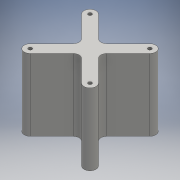
# Autodesk Inventor part: 60x60SlimSpacer
Saved by Autodesk Inventor 2016 (Build 200138000, 138)
## iProperties
Created: 2016-05-22
Part Number: 60x60SlimSpacer
Material: Generic
Document SubType Name: Modeling
Designer: Kurtis
Density: 1 g/cm^3
Appearance: Default
Author: Kurtis
Autodesk Inventor part; units mm, degrees
ref_plane "YZ Plane" through (0, 0, 0) normal (1, 0, 0) x (0, 1, 0)
ref_plane "XZ Plane" through (0, 0, 0) normal (0, 1, 0) x (-1, 0, 0)
ref_plane "XY Plane" through (0, 0, 0) normal (0, 0, 1) x (1, 0, 0)
sketch "Sketch1" plane through (0, 0, 0) normal (0, 0, 1) x (1, 0, 0)
  line L0 (-30, -30) -> (30, 30) construction
  line L1 (30, -30) -> (-30, 30) construction
  line L2 (25, 30) -> (25, 25) construction
  line L3 (-30, 30) -> (-25, 30) construction
  line L4 (-25, 30) -> (-25, 25) construction
  line L5 (-30, -25) -> (-25, -25) construction
  line L6 (30, -25) -> (25, -25) construction
  circle A0 centre (-25, 25) radius 1.5
  circle A1 centre (25, 25) radius 1.5
  circle A2 centre (25, -25) radius 1.5
  circle A3 centre (-25, -25) radius 1.5
  arc A4 (-21.4645, 28.5355) -> (-28.5355, 21.4645) centre (-25, 25) ccw
  arc A5 (28.5355, 21.4645) -> (21.4645, 28.5355) centre (25, 25) ccw
  arc A6 (21.4645, -28.5355) -> (28.5355, -21.4645) centre (25, -25) ccw
  arc A7 (-28.5355, -21.4645) -> (-21.4645, -28.5355) centre (-25, -25) ccw
  line L7 (-25, 25) -> (-30, 20) construction
  line L8 (-30, 20) -> (-20, 30) construction
  line L9 (25, 25) -> (20, 30) construction
  line L10 (30, 20) -> (25, 25) construction
  line L11 (25, -25) -> (20, -30) construction
  line L12 (20, -30) -> (30, -20) construction
  line L13 (-25, -25) -> (-20, -30) construction
  line L14 (-25, -25) -> (-30, -20) construction
  line L15 (-28.5355, -21.4645) -> (-10.6066, -3.5355)
  line L16 (3.5355, 10.6066) -> (21.4645, 28.5355)
  line L17 (-28.5355, 21.4645) -> (-10.6066, 3.5355)
  line L18 (3.5355, -10.6066) -> (21.4645, -28.5355)
  line L19 (28.5355, -21.4645) -> (10.6066, -3.5355)
  line L20 (-3.5355, 10.6066) -> (-21.4645, 28.5355)
  line L21 (-21.4645, -28.5355) -> (-3.5355, -10.6066)
  line L22 (10.6066, 3.5355) -> (28.5355, 21.4645)
  arc A8 (3.5355, -10.6066) -> (-3.5355, -10.6066) centre (0, -14.1421) ccw
  arc A9 (10.6066, 3.5355) -> (10.6066, -3.5355) centre (14.1421, 0) ccw
  arc A10 (-3.5355, 10.6066) -> (3.5355, 10.6066) centre (0, 14.1421) ccw
  arc A11 (-10.6066, -3.5355) -> (-10.6066, 3.5355) centre (-14.1421, 0) ccw
  point P0 (0, 0)
  dimension "d0" = 60
  dimension "d1" = 60
  dimension "d2" = 5
  dimension "d3" = 5
  dimension "d4" = 5
  dimension "d5" = 5
  dimension "d7" = 5
  dimension "d9" = 5
  dimension "d10" = 3
  dimension "d11" = 3
  dimension "d12" = 3
  dimension "d13" = 3
  dimension "d17" = 5
  dimension "d18" = 45
  dimension "d19" = 70.7107
  dimension "d20" = 55
  dimension "d21" = 45
  dimension "d22" = 28.2843
  dimension "d23" = 55
  dimension "d24" = 42.4264
  dimension "d25" = 28.2843
  dimension "d26" = 5
  dimension "d27" = 42.4264
  dimension "d28" = 5
  dimension "d29" = 77.7818
  constraints: 46 end point, 21 tangent, 19 point on circle, 16 point on line, 12 centre point, 8 coincident, 3 equal length, 3 equal radius, 3 perpendicular, 2 midpoint, 1 horizontal
  measures "d0" distance of L1.end L0.end
  measures "d1" distance of L0.end L1.start
  measures "d2" distance of L0.end L2.start
  measures "d3" distance of L2.start L2.end
  measures "d4" distance of L1.end L3.end
  measures "d5" distance of L3.end L4.end
  measures "d7" distance of L5.start L5.end
  measures "d9" distance of L6.start L6.end
  measures "d10" diameter of A0
  measures "d11" diameter of A1
  measures "d12" diameter of A2
  measures "d13" diameter of A3
  measures "d17" radius of A8
  measures "d18" angle of L5 L10
  measures "d19" distance between parallel lines of L10 L14
  measures "d20" distance between parallel lines of L6 L3
  measures "d21" distance from line of L10.start L6
  measures "d22" distance from line of L12.end L10
  measures "d23" distance from line of L9.end L6
  measures "d24" distance from line of L11.end L10
  measures "d25" distance from line of L8.end L10
  measures "d26" distance from line of L13.end L6
  measures "d27" distance from line of L7.end L10
  measures "d28" distance from line of L14.end L6
  measures "d29" distance from line of L0.start L10
extrude "Main Body" add sketch "Sketch1" along normal blind 60
body "Solid2"
